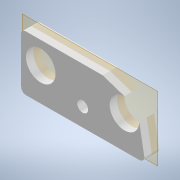
# Autodesk Inventor part: srodek
Saved by Autodesk Inventor 2022.3 (Build 263350000, 350)
## iProperties
Created: 2022-12-14
Part Number: srodek
Material: Generic
Document SubType Name: Modeling
Designer: komputer
Density: 1 g/cm^3
Appearance: Default
Author: komputer
Autodesk Inventor part; units mm, degrees
ref_plane "YZ Plane" through (0, 0, 0) normal (1, 0, 0) x (0, 1, 0)
ref_plane "XZ Plane" through (0, 0, 0) normal (0, 1, 0) x (-1, 0, 0)
ref_plane "XY Plane" through (0, 0, 0) normal (0, 0, 1) x (1, 0, 0)
ref_plane "Work Plane1" through (1.0737, -2.7207, -1.3848) normal (0, 0, 1) x (1, 0.0049, 0)
sketch "Sketch1" plane through (1.0737, -2.7207, -1.3848) normal (0, 0, 1) x (1, 0.0049, 0)
  line L0 (-12.5, -4.85) -> (-12.5, 4.35) projected
  line L1 (12.5, 4.35) -> (12.5, -4.85) projected
  line L2 (11.5, -5.85) -> (-11.5, -5.85) projected
  circle A0 centre (8.5, 0.85) radius 3 projected
  circle A1 centre (-8.5, 0.85) radius 3 projected
  circle A2 centre (0, -2.15) radius 1.1
  line L3 (4.0694, -5.85) -> (-4.0694, -5.85)
  circle A3 centre (0, -2.15) radius 1.1 projected
  line L4 (-11.5, 5.35) -> (11.5, 5.35) projected
  arc A4 (-12.5, -4.85) -> (-11.5, -5.85) centre (-11.5, -4.85) ccw projected
  arc A5 (-11.5, 5.35) -> (-12.5, 4.35) centre (-11.5, 4.35) ccw projected
  arc A6 (12.5, 4.35) -> (11.5, 5.35) centre (11.5, 4.35) ccw projected
  arc A7 (11.5, -5.85) -> (12.5, -4.85) centre (11.5, -4.85) ccw projected
  point P0 (-1.0602, 2.726)
  dimension "d0" = 2.2
  constraints: 2 end point, 1 centre point, 1 horizontal
  measures "d0" diameter of A2
extrude "Extrusion1" add sketch "Sketch1" along normal mid plane 4
sketch "Sketch2" plane through (1.0737, -2.7207, 0.6152) normal (0, 0, 1) x (1, 0.0049, 0)
  line L0 (-12.5, 4.35) -> (-12.5, -4.85) projected
  line L1 (-11.5, -5.85) -> (11.5, -5.85) projected
  line L2 (12.5, -4.85) -> (12.5, 4.35) projected
  circle A0 centre (8.5, 0.85) radius 3 projected
  circle A1 centre (-8.5, 0.85) radius 3 projected
  line L3 (11.5, 0.85) -> (12.5, 0.85)
  line L4 (12.5, -4.85) -> (12.5, 4.35) projected
  circle A2 centre (8.5, 0.85) radius 3 projected
  line L5 (8.5, 3.85) -> (0.045, 5.85)
  line L6 (12.5, 5.85) -> (-12.5, 5.85) projected
  circle A3 centre (0, -2.15) radius 1.1 projected
  line L7 (11.5, 5.35) -> (-11.5, 5.35) projected
  arc A4 (-12.5, -4.85) -> (-11.5, -5.85) centre (-11.5, -4.85) ccw projected
  arc A5 (11.5, -5.85) -> (12.5, -4.85) centre (11.5, -4.85) ccw projected
  arc A6 (12.5, 4.35) -> (11.5, 5.35) centre (11.5, 4.35) ccw projected
  arc A7 (-11.5, 5.35) -> (-12.5, 4.35) centre (-11.5, 4.35) ccw projected
  point P0 (-1.0602, 2.726)
  point P1 (-12.5, 5.85)
  point P2 (8.5, 3.85)
  point P3 (12.5, 0.85)
  constraints: 4 end point, 1 perpendicular, 1 point on circle, 1 point on line, 4 other
extrude "Extrusion2" [suppressed]
sketch "Sketch3" plane through (1.0737, -2.7207, 0.6152) normal (0, 0, 1) x (1, 0.0049, 0)
  line L0 (-12.5, 4.35) -> (-12.5, -4.85) projected
  line L1 (-11.5, -5.85) -> (11.5, -5.85) projected
  line L2 (12.5, -4.85) -> (12.5, 4.35) projected
  circle A0 centre (8.5, 0.85) radius 3 projected
  circle A1 centre (-8.5, 0.85) radius 3 projected
  circle A2 centre (0, -2.15) radius 1.1 projected
  line L3 (-12.5, 4.35) -> (-12.5, -4.85) projected
  line L4 (-12.5, 5.85) -> (-9.6209, 5.85)
  line L5 (-9.6209, 5.85) -> (-9.6209, 5.35)
  line L6 (-9.6209, 5.35) -> (-12.5, 5.35)
  line L7 (-12.5, 5.35) -> (-12.5, 5.85)
  line L8 (-12.5, 5.85) -> (7.0362, 5.85)
  line L9 (7.0362, 5.85) -> (7.0362, 5.35)
  line L10 (7.0362, 5.35) -> (-12.5, 5.35)
  line L11 (-12.5, 5.35) -> (-12.5, 5.85)
  arc A3 (12.5, 4.35) -> (11.5, 5.35) centre (11.5, 4.35) ccw projected
  line L12 (11.5, 5.35) -> (-11.5, 5.35) projected
  arc A4 (-11.5, 5.35) -> (-12.5, 4.35) centre (-11.5, 4.35) ccw projected
  arc A5 (-12.5, -4.85) -> (-11.5, -5.85) centre (-11.5, -4.85) ccw projected
  arc A6 (11.5, -5.85) -> (12.5, -4.85) centre (11.5, -4.85) ccw projected
  point P0 (-1.0602, 2.726)
  point P1 (-12.5, -5.85)
  point P2 (-12.5, 5.35)
  point P3 (-9.6209, 5.35)
  point P4 (-11.5, 5.35)
  point P5 (-12.5, 5.35)
  point P6 (-9.6209, 5.35)
  point P7 (7.0362, 5.35)
  point P8 (7.0362, 5.35)
  dimension "d5" = 0.5
  constraints: 16 end point, 4 parallel, 2 horizontal, 2 perpendicular, 1 point on line
  measures "d5" distance of L4.end L5.end
extrude "Extrusion3" cut sketch "Sketch3" against normal blind 10 contours A4 L6 L10 L12 A3 L2 A6 L1 A5 L0 | L6 L7 L4 L5 | L5 L8 L9 L10 | A1 | A2
sketch "Sketch4" plane through (1.0737, -2.7207, -1.3848) normal (0, 0, 1) x (1, 0.0049, 0)
  arc A0 (-12.5, -4.85) -> (-11.5, -5.85) centre (-11.5, -4.85) ccw projected
  line L0 (-11.5, -5.85) -> (11.5, -5.85) projected
  arc A1 (11.5, -5.85) -> (12.5, -4.85) centre (11.5, -4.85) ccw projected
  line L1 (12.5, -4.85) -> (12.5, 4.35) projected
  arc A2 (12.5, 4.35) -> (11.5, 5.35) centre (11.5, 4.35) ccw projected
  line L2 (11.5, 5.35) -> (-11.5, 5.35) projected
  arc A3 (-11.5, 5.35) -> (-12.5, 4.35) centre (-11.5, 4.35) ccw projected
  line L3 (-12.5, 4.35) -> (-12.5, -4.85) projected
  circle A4 centre (0, -2.15) radius 1.1 projected
  circle A5 centre (8.5, 0.85) radius 3 projected
  circle A6 centre (-8.5, 0.85) radius 3 projected
  line L4 (8.5, 3.85) -> (4.0971, 5.35)
  line L5 (11.5, 0.85) -> (12.5, -4.85)
  point P0 (-1.0602, 2.726)
  constraints: 4 end point, 2 point on circle, 1 point on line
extrude "Extrusion4" add sketch "Sketch4" along normal mid plane 3 contours L3 A3 L2 L4 A5 L5 A1 L0 A0
body "Solid1"
